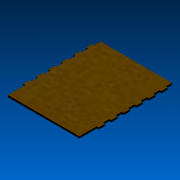
# Autodesk Inventor part: Avant
Saved by Autodesk Inventor 2013 SP2 (Build 170200200, 200)
## iProperties
Created: 2015-09-15
Part Number: Avant
Material: Generic
Document SubType Name: Modeling
Designer: jeanfrancois
Density: 1 g/cm^3
Author: jeanfrancois
Autodesk Inventor part; units mm, degrees
ref_plane "YZ Plane" through (0, 0, 0) normal (1, 0, 0) x (0, 1, 0)
ref_plane "XZ Plane" through (0, 0, 0) normal (0, 1, 0) x (-1, 0, 0)
ref_plane "XY Plane" through (0, 0, 0) normal (0, 0, 1) x (1, 0, 0)
sketch "Esquisse1" plane through (0, 0, 0) normal (0, 0, 1) x (1, 0, 0)
  line L0 (46.7128, 20.0366) -> (46.7128, 10.0366)
  line L1 (49.7128, 30.0366) -> (49.7128, 20.0366)
  line L2 (46.7128, 40.0366) -> (46.7128, 30.0366)
  line L3 (49.7128, 50.0366) -> (49.7128, 40.0366)
  line L4 (46.7128, 10.0366) -> (49.7128, 10.0366)
  line L5 (46.7128, 20.0366) -> (49.7128, 20.0366)
  line L6 (46.7128, 30.0366) -> (49.7128, 30.0366)
  line L7 (46.7128, 60.0366) -> (46.7128, 50.0366)
  line L8 (-67.2872, 20.0366) -> (-67.2872, 10.0366)
  line L9 (-67.2872, 20.0366) -> (-70.2872, 20.0366)
  line L10 (-70.2872, 30.0366) -> (-70.2872, 20.0366)
  line L11 (-67.2872, 30.0366) -> (-70.2872, 30.0366)
  line L12 (-67.2872, 40.0366) -> (-67.2872, 30.0366)
  line L13 (-67.2872, 40.0366) -> (-70.2872, 40.0366)
  line L14 (-70.2872, 50.0366) -> (-70.2872, 40.0366)
  line L15 (-67.2872, 50.0366) -> (-70.2872, 50.0366)
  line L16 (-67.2872, 60.0366) -> (-67.2872, 50.0366)
  line L17 (-67.2872, 60.0366) -> (-70.2872, 60.0366)
  line L18 (-70.2872, 70.0366) -> (-70.2872, 60.0366)
  line L19 (-67.2872, 70.0366) -> (-70.2872, 70.0366)
  line L20 (-67.2872, 80.0366) -> (-67.2872, 70.0366)
  line L21 (46.7128, 40.0366) -> (49.7128, 40.0366)
  line L22 (46.7128, 50.0366) -> (49.7128, 50.0366)
  line L23 (46.7128, 60.0366) -> (49.7128, 60.0366)
  line L24 (49.7128, 70.0366) -> (49.7128, 60.0366)
  line L25 (46.7128, 70.0366) -> (49.7128, 70.0366)
  line L26 (46.7128, 80.0366) -> (46.7128, 70.0366)
  line L27 (46.7128, 80.0366) -> (-67.2872, 80.0366)
  line L28 (46.7128, -39.9634) -> (46.7128, -67.6814)
  line L29 (49.7128, -29.9634) -> (49.7128, -39.9634)
  line L30 (46.7128, -19.9634) -> (46.7128, -29.9634)
  line L31 (49.7128, -9.9634) -> (49.7128, -19.9634)
  line L32 (46.7128, 0.0366) -> (46.7128, -9.9634)
  line L33 (49.7128, 10.0366) -> (49.7128, 0.0366)
  line L34 (46.7128, -39.9634) -> (49.7128, -39.9634)
  line L35 (46.7128, -29.9634) -> (49.7128, -29.9634)
  line L36 (46.7128, -19.9634) -> (49.7128, -19.9634)
  line L37 (46.7128, -9.9634) -> (49.7128, -9.9634)
  line L38 (46.7128, 0.0366) -> (49.7128, 0.0366)
  line L39 (-70.2872, 10.0366) -> (-70.2872, 0.0366)
  line L40 (-67.2872, 0.0366) -> (-70.2872, 0.0366)
  line L41 (-67.2872, 0.0366) -> (-67.2872, -9.9634)
  line L42 (-67.2872, -9.9634) -> (-70.2872, -9.9634)
  line L43 (-67.2872, -67.6814) -> (46.7128, -67.6814)
  line L44 (-70.2872, -9.9634) -> (-70.2872, -19.9634)
  line L45 (-67.2872, -19.9634) -> (-70.2872, -19.9634)
  line L46 (-67.2872, -19.9634) -> (-67.2872, -29.9634)
  line L47 (-67.2872, -29.9634) -> (-70.2872, -29.9634)
  line L48 (-70.2872, -29.9634) -> (-70.2872, -39.9634)
  line L49 (-67.2872, -39.9634) -> (-70.2872, -39.9634)
  line L50 (-67.2872, -39.9634) -> (-67.2872, -67.6814)
  line L51 (-67.2872, 10.0366) -> (-70.2872, 10.0366)
  point P0 (0, 0)
  constraints: 104 end point
extrude "Extrusion1" add sketch "Esquisse1" along normal blind 3
